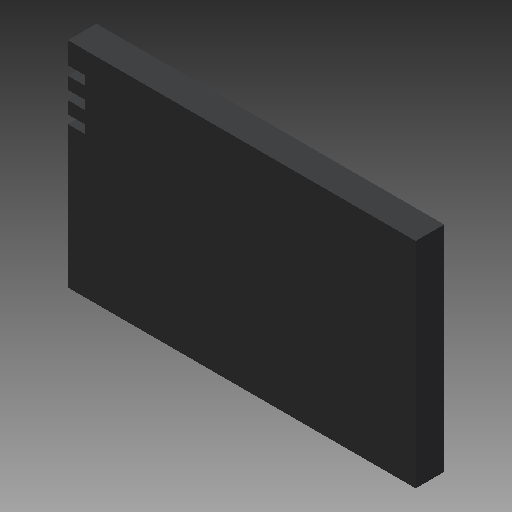
# Autodesk Inventor part: bateria
Saved by Autodesk Inventor 2017 (Build 210142000, 142)
## iProperties
Created: 2016-09-09
Part Number: bateria
Material: Generic
Document SubType Name: Modeling
Designer: Paulo Loma
Density: 1 g/cm^3
Appearance: Generic
Author: Paulo Loma
Autodesk Inventor part; units mm, degrees
ref_plane "YZ Plane" through (0, 0, 0) normal (1, 0, 0) x (0, 1, 0)
ref_plane "XZ Plane" through (0, 0, 0) normal (0, 1, 0) x (-1, 0, 0)
ref_plane "XY Plane" through (0, 0, 0) normal (0, 0, 1) x (1, 0, 0)
sketch "Sketch1" plane through (0, 0, 0) normal (0, 0, 1) x (1, 0, 0)
  line L0 (-31.1, -19.15) -> (31.1, -19.15)
  line L1 (31.1, -19.15) -> (31.1, 19.15)
  line L2 (31.1, 19.15) -> (-31.1, 19.15)
  line L3 (-31.1, 19.15) -> (-31.1, -19.15)
  line L4 (-31.1, -19.15) -> (31.1, 19.15) construction
  line L5 (31.1, -19.15) -> (-31.1, 19.15) construction
  point P0 (0, 0)
  dimension "d0" = 38.3
  dimension "d1" = 62.2
  constraints: 12 end point, 2 midpoint, 2 parallel, 1 horizontal, 1 perpendicular
  measures "d0" distance of L0.end L1.end
  measures "d1" distance of L1.end L2.end
extrude "Extrusion1" add sketch "Sketch1" along normal blind 5.1
sketch "Sketch2" plane through (0, 0, 5.1) normal (0, 0, 1) x (1, 0, 0)
  line L0 (-31.1, 19.15) -> (-28.1, 19.15)
  line L1 (-28.1, 19.15) -> (-28.1, 6.15)
  line L2 (-28.1, 6.15) -> (-31.1, 6.15)
  line L3 (-31.1, 6.15) -> (-31.1, 19.15)
  line L4 (-31.1, 19.15) -> (-31.1, 15.25)
  line L5 (-31.1, 19.15) -> (-31.1, -19.15) projected
  line L6 (-31.1, 15.25) -> (-28.1, 15.25)
  line L7 (-31.1, 15.25) -> (-31.1, 13.65)
  line L8 (-31.1, 13.65) -> (-28.1, 13.65)
  line L9 (-31.1, 13.65) -> (-31.1, 11.45)
  line L10 (-31.1, 11.45) -> (-28.1, 11.45)
  line L11 (-31.1, 11.45) -> (-31.1, 9.85)
  line L12 (-31.1, 9.85) -> (-28.1, 9.85)
  line L13 (-31.1, 9.85) -> (-31.1, 7.65)
  line L14 (-31.1, 7.65) -> (-28.1, 7.65)
  point P0 (0, 0)
  dimension "d4" = 13
  dimension "d5" = 3
  dimension "d6" = 3.9
  dimension "d7" = 1.6
  dimension "d8" = 2.2
  dimension "d9" = 1.6
  dimension "d10" = 2.2
  constraints: 28 end point, 10 point on line, 6 perpendicular, 2 parallel, 1 horizontal
  measures "d4" distance of L0.end L1.end
  measures "d5" distance of L1.end L2.end
  measures "d6" distance of L0.start L4.end
  measures "d7" distance of L4.end L7.end
  measures "d8" distance of L7.end L9.end
  measures "d9" distance of L9.end L11.end
  measures "d10" distance of L11.end L13.end
extrude "Extrusion2" cut sketch "Sketch2" against normal blind 3.6 contours L6 L1 L8 L3 | L10 L1 L12 L3 | L14 L1 L2 L3
body "Solid1"
